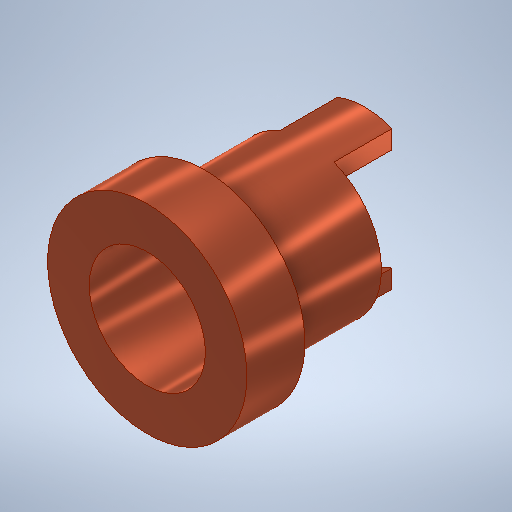
# Autodesk Inventor part: TR8_AntiBacklashNutSecondary
Saved by Autodesk Inventor 2025.2 (Build 292293000, 293)
## iProperties
Created: 2017-03-01
Part Number: TR8_AntiBacklashNutSecondary
Material: Ogólny
Document SubType Name: Modeling
Designer: user
Density: 1 g/cm^3
Appearance: Gorący metal 1400F
Author: user
Autodesk Inventor part; units mm, degrees
ref_plane "XZ Plane" through (0, 0, 0) normal (0, 1, 0) x (-1, 0, 0)
ref_plane "XY Plane" through (0, 0, 0) normal (0, 0, 1) x (1, 0, 0)
sketch "Szkic1" plane through (0, 0, 0) normal (0, 1, 0) x (-1, 0, 0)
  circle A0 centre (0, 0) radius 6.875
  circle A1 centre (0, 0) radius 4
  dimension "d0" = 13.75
  dimension "d1" = 8
  constraints: 2 centre point, 2 coincident
  measures "d0" diameter of A0
  measures "d1" diameter of A1
extrude "Wyciągnięcie proste1" add sketch "Szkic1" along normal blind 4
sketch "Szkic2" plane through (0, 4, 0) normal (0, 1, 0) x (1, 0, 0)
  circle A0 centre (0, 0) radius 5.15
  circle A1 centre (0, 0) radius 4 projected
  dimension "d4" = 10.3
  constraints: 1 centre point, 1 coincident
  measures "d4" diameter of A0
extrude "Wyciągnięcie proste2" add sketch "Szkic2" along normal blind 11
ref_plane "Płaszczyzna konstrukcyjna1" through (1.875, 0, 0) normal (1, 0, 0) x (0, 1, 0)
sketch "Szkic3" plane through (1.875, 0, 0) normal (1, 0, 0) x (0, 1, 0)
  line L0 (15, 4) -> (15, -4) projected
  line L1 (0, -4) -> (0, 4) projected
  line L2 (4, 5.15) -> (15, 5.15) projected
  line L3 (4, -5.15) -> (15, -5.15) projected
  line L4 (15, -5.15) -> (15, 5.15) projected
  line L5 (15, 5.15) -> (11, 5.15)
  line L6 (11, 5.15) -> (11, -5.15)
  line L7 (11, -5.15) -> (15, -5.15)
  line L8 (15, -5.15) -> (15, 5.15)
  point P0 (0, 0)
  dimension "d8" = 4
  constraints: 8 end point, 2 parallel, 1 horizontal, 1 perpendicular, 1 point on line
  measures "d8" distance of L7.end L6.end
extrude "Wyciągnięcie proste3" cut sketch "Szkic3" along normal through all
ref_plane "Płaszczyzna konstrukcyjna2" through (-1.875, 0, 0) normal (1, 0, 0) x (0, 1, 0)
sketch "Szkic4" plane through (-1.875, 0, 0) normal (1, 0, 0) x (0, 1, 0)
  line L0 (4, 5.15) -> (4, -5.15) projected
  line L1 (15, -4.7965) -> (11, -4.7965) projected
  line L2 (11, -4.7965) -> (11, 4.7965) projected
  line L3 (11, 4.7965) -> (15, 4.7965) projected
  line L4 (15, -4.7965) -> (15, 4.7965) projected
  line L5 (4, 5.15) -> (15, 5.15) projected
  line L6 (15, -6.2367) -> (11, -6.2367)
  line L7 (11, -6.2367) -> (11, 6.0914)
  line L8 (11, 6.0914) -> (15, 6.0914)
  line L9 (15, 6.0914) -> (15, -6.2367)
  point P0 (0, 0)
  constraints: 8 end point, 2 parallel, 1 horizontal, 1 perpendicular
extrude "Wyciągnięcie proste4" cut sketch "Szkic4" against normal through all
